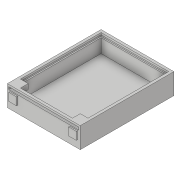
# Autodesk Inventor part: Electronics Container
Saved by Autodesk Inventor 2018.3 (Build 223284000, 284)
## iProperties
Created: 2019-01-09
Part Number: Electronics Container
Material: Generic
Document SubType Name: Modeling
Designer: aye06091
Mass: 59.0991 g
Surface Area: 408.467 cm^2
Volume: 59.0991 cm^3
Density: 1 g/cm^3
Appearance: Default
Author: aye06091
Autodesk Inventor part; units mm, degrees
ref_plane "YZ Plane" through (0, 0, 0) normal (1, 0, 0) x (0, 1, 0)
ref_plane "XZ Plane" through (0, 0, 0) normal (0, 1, 0) x (-1, 0, 0)
ref_plane "XY Plane" through (0, 0, 0) normal (0, 0, 1) x (1, 0, 0)
sketch "Sketch1" plane through (0, 0, 0) normal (0, 0, 1) x (1, 0, 0)
  line L0 (0, 0) -> (88.9, 0)
  line L1 (88.9, 0) -> (88.9, -25.4)
  line L2 (88.9, -25.4) -> (0, -25.4)
  line L3 (0, -25.4) -> (0, 0)
  dimension "d0" = 88.9
  dimension "d1" = 25.4
  constraints: 8 end point, 2 parallel, 1 horizontal, 1 perpendicular
  measures "d0" distance of L1.end L2.end
  measures "d1" distance of L2.end L0.start
extrude "Extrusion1" add sketch "Sketch1" against normal blind 114.3
sketch "Sketch2" plane through (0, 0, 0) normal (0, 1, 0) x (1, 0, 0)
  line L0 (0, 0) -> (88.9, 0) projected
  line L1 (88.9, 0) -> (88.9, 114.3) projected
  line L2 (0, 114.3) -> (88.9, 114.3) projected
  line L3 (0, 0) -> (0, 114.3) projected
  line L4 (3.175, 3.175) -> (85.725, 3.175)
  line L5 (85.725, 3.175) -> (85.725, 111.125)
  line L6 (85.725, 111.125) -> (3.175, 111.125)
  line L7 (3.175, 111.125) -> (3.175, 3.175)
  dimension "d4" = 3.175
  dimension "d5" = 3.175
  dimension "d6" = 3.175
  dimension "d7" = 3.175
  constraints: 8 end point, 2 parallel, 1 horizontal, 1 perpendicular
  measures "d4" distance between parallel lines of L3 L7
  measures "d5" distance between parallel lines of L0 L4
  measures "d6" distance between parallel lines of L1 L5
  measures "d7" distance between parallel lines of L2 L6
extrude "Extrusion2" cut sketch "Sketch2" against normal blind 22.225 contours L7 L6 L5 L4
sketch "Sketch3" plane through (0, 0, 0) normal (0, 0, 1) x (1, 0, 0)
  line L0 (0, -25.4) -> (0, 0) projected
  line L1 (88.9, 0) -> (88.9, -25.4) projected
  line L2 (0, -25.4) -> (0, 0) projected
  line L3 (88.9, 0) -> (88.9, -25.4) projected
  line L4 (1.5875, -2.3041) -> (87.3125, -2.3041)
  line L5 (87.3125, -2.3041) -> (87.3125, -5.4791)
  line L6 (87.3125, -5.4791) -> (1.5875, -5.4791)
  line L7 (1.5875, -5.4791) -> (1.5875, -2.3041)
  dimension "d46" = 3.175
  dimension "d47" = 1.5875
  dimension "d49" = 1.5875
  constraints: 8 end point, 2 parallel, 1 horizontal, 1 perpendicular
  measures "d46" distance between parallel lines of L6 L4
  measures "d47" distance between parallel lines of L0 L7
  measures "d49" distance between parallel lines of L1 L5
extrude "Extrusion3" cut sketch "Sketch3" against normal blind 112.7125
sketch "Sketch5" plane through (0, 0, 0) normal (0, 1, 0) x (1, 0, 0)
  line L0 (3.175, 3.175) -> (3.175, 111.125) projected
  line L1 (3.175, 3.175) -> (12.7, 3.175)
  line L2 (12.7, 3.175) -> (12.7, 12.7)
  line L3 (12.7, 12.7) -> (3.175, 12.7)
  line L4 (3.175, 12.7) -> (3.175, 3.175)
  line L5 (85.725, 3.175) -> (76.2, 3.175)
  line L6 (76.2, 3.175) -> (76.2, 12.7)
  line L7 (76.2, 12.7) -> (85.725, 12.7)
  line L8 (85.725, 12.7) -> (85.725, 3.175)
  dimension "d64" = 9.525
  dimension "d67" = 9.525
  dimension "d68" = 9.525
  dimension "d69" = 9.525
  constraints: 16 end point, 4 parallel, 2 horizontal, 2 perpendicular
  measures "d64" distance of L6.end L7.end
  measures "d67" distance of L2.end L3.end
  measures "d68" distance of L1.end L2.end
  measures "d69" distance of L5.end L6.end
extrude "Extrusion4" add sketch "Sketch5" against normal blind 6.35
sketch "Sketch6" plane through (0, 0, 0) normal (0, 0, 1) x (1, 0, 0)
  line L0 (12.7, -6.7991) -> (3.175, -6.7991)
  line L1 (3.175, -6.7991) -> (3.175, -16.3241)
  line L2 (3.175, -16.3241) -> (12.7, -16.3241)
  line L3 (12.7, -16.3241) -> (12.7, -6.7991)
  line L4 (76.2, -6.7991) -> (85.725, -6.7991)
  line L5 (85.725, -6.7991) -> (85.725, -16.3241)
  line L6 (85.725, -16.3241) -> (76.2, -16.3241)
  line L7 (76.2, -16.3241) -> (76.2, -6.7991)
  line L8 (87.3125, -5.4791) -> (1.5875, -5.4791) projected
  line L9 (0, -25.4) -> (0, 0) projected
  line L10 (88.9, 0) -> (88.9, -25.4) projected
  dimension "d70" = 9.525
  dimension "d71" = 9.525
  dimension "d72" = 9.525
  dimension "d73" = 9.525
  dimension "d76" = 1.32
  dimension "d77" = 1.32
  dimension "d78" = 3.175
  dimension "d79" = 3.175
  constraints: 16 end point, 4 parallel, 2 horizontal, 2 perpendicular, 2 point on line
  measures "d70" distance of L0.start L0.end
  measures "d71" distance of L2.end L0.start
  measures "d72" distance of L6.end L4.start
  measures "d73" distance of L4.start L4.end
  measures "d76" distance between parallel lines of L8 L0
  measures "d77" distance between parallel lines of L8 L4
  measures "d78" distance between parallel lines of L9 L1
  measures "d79" distance between parallel lines of L10 L5
extrude "Extrusion5" add sketch "Sketch6" along normal blind 1.5875
equation "\"d49\" = d47"
equation "\"d65\" = d62"
equation "\"d73\" = d71"
equation "\"d79\" = d78"
equation "\"d62\" = 6.35"
body "Solid1"
